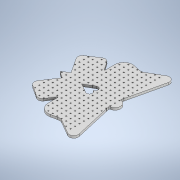
# Autodesk Inventor part: Butterfly(my own.3)
Saved by Autodesk Inventor 2020.2 (Build 242310000, 310)
## iProperties
Created: 2020-02-15
Part Number: Butterfly(my own.3)
Material: Generic
Document SubType Name: Modeling
Designer: lenovo
Density: 1 g/cm^3
Appearance: Default
Author: lenovo
Autodesk Inventor part; units mm, degrees
ref_plane "YZ Plane" through (0, 0, 0) normal (1, 0, 0) x (0, 1, 0)
ref_plane "XZ Plane" through (0, 0, 0) normal (0, 1, 0) x (-1, 0, 0)
ref_plane "XY Plane" through (0, 0, 0) normal (0, 0, 1) x (1, 0, 0)
sketch "Sketch1" plane through (0, 0, 0) normal (0, 1, 0) x (-1, 0, 0)
  line L0 (22.8541, 0.8351) -> (9.6752, 9.5184)
  line L1 (24.1214, 0.0001) -> (39.9037, 0.0001) construction
  line L2 (9.3904, 10.9036) -> (30.8478, 43.4702)
  line L3 (27.9993, 57.3225) -> (2.9481, 73.8281)
  line L4 (-10.9042, 70.9796) -> (-22.8239, 52.8887)
  line L5 (-24.659, 53.4389) -> (-24.659, 85.1036)
  line L6 (-24.659, 85.1036) -> (-24.659, 75.1841)
  line L7 (-48.9878, 94.7101) -> (-62.9353, 91.618)
  line L8 (-73.6103, 93.261) -> (-105.0047, 111.3865)
  line L9 (-119.7515, 100.4904) -> (-99.9709, 14.2618)
  line L10 (-124.8839, 122.8638) -> (0.9973, 122.8638) construction
  arc A0 (-101.2792, 12.4343) -> (-112.4983, 0.0001) centre (-99.9983, 0.0001) ccw
  line L11 (40, 0.0001) -> (-130, 0.0001)
  line L12 (22.8541, -0.8349) -> (9.6752, -9.5182)
  line L13 (9.3904, -10.9034) -> (30.8478, -43.47)
  line L14 (27.9993, -57.3223) -> (2.9481, -73.8279)
  line L15 (-10.9042, -70.9794) -> (-22.8239, -52.8885)
  line L16 (-24.659, -53.4387) -> (-24.659, -85.1034)
  line L17 (-24.659, -85.1034) -> (-24.659, -75.1839)
  line L18 (-48.9878, -94.7099) -> (-62.9353, -91.6178)
  line L19 (-73.6103, -93.2608) -> (-105.0047, -111.3864)
  line L20 (-119.7515, -100.4902) -> (-99.9709, -14.2616)
  arc A1 (-112.4983, 0.0001) -> (-101.2792, -12.4341) centre (-99.9983, 0.0001) ccw
  arc A2 (30.8478, 43.4702) -> (27.9993, 57.3225) centre (22.4974, 48.9721) ccw
  arc A3 (2.9481, 73.8281) -> (-10.9042, 70.9796) centre (-2.5538, 65.4777) ccw
  arc A4 (27.9993, -57.3223) -> (30.8478, -43.47) centre (22.4974, -48.9719) ccw
  arc A5 (-10.9042, -70.9794) -> (2.9481, -73.8279) centre (-2.5538, -65.4775) ccw
  arc A6 (-24.659, 53.4389) -> (-22.8239, 52.8887) centre (-23.659, 53.4389) ccw
  arc A7 (-22.8239, -52.8885) -> (-24.659, -53.4387) centre (-23.659, -53.4387) ccw
  arc A8 (9.3904, 10.9036) -> (9.6752, 9.5184) centre (10.2254, 10.3534) ccw
  arc A9 (9.6752, -9.5182) -> (9.3904, -10.9034) centre (10.2254, -10.3532) ccw
  arc A10 (22.8541, -0.8349) -> (22.8541, 0.8351) centre (22.3039, 0.0001) ccw
  arc A11 (-24.659, 75.1841) -> (-48.9878, 94.7101) centre (-44.659, 75.1841) ccw
  arc A12 (-48.9878, -94.7099) -> (-24.659, -75.1839) centre (-44.659, -75.1839) ccw
  arc A13 (-105.0047, 111.3865) -> (-119.7515, 100.4904) centre (-110.0047, 102.7263) ccw
  arc A14 (-119.7515, -100.4902) -> (-105.0047, -111.3864) centre (-110.0047, -102.7261) ccw
  arc A15 (-73.6103, 93.261) -> (-62.9353, 91.618) centre (-66.1603, 106.1648) ccw
  arc A16 (-62.9353, -91.6178) -> (-73.6103, -93.2608) centre (-66.1603, -106.1646) ccw
  arc A17 (-101.2792, 12.4343) -> (-99.9709, 14.2618) centre (-101.4329, 13.9264) ccw
  arc A18 (-99.9709, -14.2616) -> (-101.2792, -12.4341) centre (-101.4329, -13.9262) ccw
  point P0 (0, 0)
  point P1 (8.8402, 10.0686)
  point P2 (36.3497, 51.8206)
  point P3 (-5.4023, 79.33)
  point P4 (-24.659, 50.1036)
  point P5 (-24.659, 100.1036)
  point P6 (-68.5923, 90.3638)
  point P7 (-99.565, 12.4926)
  point P8 (8.8402, -10.0684)
  point P9 (36.3497, -51.8204)
  point P10 (-5.4023, -79.3298)
  point P11 (-24.659, -50.1034)
  point P12 (-24.659, -100.1034)
  point P13 (-68.5923, -90.3636)
  point P14 (-124.8839, -122.8636)
  point P15 (-99.565, -12.4924)
  dimension "d0" = 18.3
  dimension "d1" = 146.62
  dimension "d2" = 50
  dimension "d3" = 90
  dimension "d4" = 50
  dimension "d5" = 90
  dimension "d6" = 35
  dimension "d7" = 90
  dimension "d8" = 35
  dimension "d9" = 15
  dimension "d10" = 45
  dimension "d11" = 77.5
  dimension "d12" = 65
  dimension "d13" = 137.5
  dimension "d14" = 77.08
  dimension "d15" = 25
  dimension "d16" = 170
  dimension "d17" = 10
  dimension "d18" = 1
  dimension "d19" = 20
  dimension "d20" = 14.9
  dimension "d21" = 1.5
  constraints: 42 end point, 40 point on circle, 37 point on line, 34 tangent, 19 centre point, 12 equal radius, 9 symmetric about line, 3 perpendicular, 2 horizontal, 1 equal length, 1 vertical, 1 other
  measures "d0" distance of L1.start point (8.84, 10.069)
  measures "d1" angle of L1 L0
  measures "d2" distance of point (8.84, 10.069) point (36.35, 51.821)
  measures "d3" angle of L0 L2
  measures "d4" distance of point (36.35, 51.821) point (-5.402, 79.33)
  measures "d5" angle of L3 L2
  measures "d6" distance of point (-5.402, 79.33) point (-24.659, 50.104)
  measures "d7" angle of L4 L3
  measures "d8" distance of point (-24.659, 50.104) L5.end
  measures "d9" distance of L5.end point (-24.659, 100.104)
  measures "d10" distance of point (-24.659, 100.104) point (-68.592, 90.364)
  measures "d11" angle of L7 L6
  measures "d12" distance of point (-68.592, 90.364) L10.start
  measures "d13" angle of L7 L8
  measures "d14" angle of L9 L10
  measures "d15" diameter of A0
  measures "d16" distance of L11.start L11.end
  measures "d17" radius of A2
  measures "d18" radius of A6
  measures "d19" radius of A11
  measures "d20" radius of A15
  measures "d21" radius of A17
extrude "Extrusion1" add sketch "Sketch1" along normal blind 5
sketch "Sketch2" plane through (0, 5, 0) normal (0, 1, 0) x (1, 0, 0)
  line L0 (-1, -1) -> (1, -1)
  line L1 (1, -1) -> (1, 1)
  line L2 (1, 1) -> (-1, 1)
  line L3 (-1, 1) -> (-1, -1)
  line L4 (-1, -1) -> (1, 1) construction
  line L5 (1, -1) -> (-1, 1) construction
  line L6 (-55, 0) -> (141.5585, 0)
  line L7 (0, 115) -> (0, -134.2875)
  line L8 (11, 1) -> (9, 1)
  line L9 (9, 1) -> (9, -1)
  line L10 (11, -1) -> (11, 1)
  line L11 (9, -1) -> (11, -1)
  line L12 (21, 1) -> (19, 1)
  line L13 (19, 1) -> (19, -1)
  line L14 (21, -1) -> (21, 1)
  line L15 (19, -1) -> (21, -1)
  line L16 (31, 1) -> (29, 1)
  line L17 (29, 1) -> (29, -1)
  line L18 (31, -1) -> (31, 1)
  line L19 (29, -1) -> (31, -1)
  line L20 (41, 1) -> (39, 1)
  line L21 (39, 1) -> (39, -1)
  line L22 (41, -1) -> (41, 1)
  line L23 (39, -1) -> (41, -1)
  line L24 (51, 1) -> (49, 1)
  line L25 (49, 1) -> (49, -1)
  line L26 (51, -1) -> (51, 1)
  line L27 (49, -1) -> (51, -1)
  line L28 (61, 1) -> (59, 1)
  line L29 (59, 1) -> (59, -1)
  line L30 (61, -1) -> (61, 1)
  line L31 (59, -1) -> (61, -1)
  line L32 (71, 1) -> (69, 1)
  line L33 (69, 1) -> (69, -1)
  line L34 (71, -1) -> (71, 1)
  line L35 (69, -1) -> (71, -1)
  line L36 (81, 1) -> (79, 1)
  line L37 (79, 1) -> (79, -1)
  line L38 (81, -1) -> (81, 1)
  line L39 (79, -1) -> (81, -1)
  line L40 (91, 1) -> (89, 1)
  line L41 (89, 1) -> (89, -1)
  line L42 (91, -1) -> (91, 1)
  line L43 (89, -1) -> (91, -1)
  line L44 (101, 1) -> (99, 1)
  line L45 (99, 1) -> (99, -1)
  line L46 (101, -1) -> (101, 1)
  line L47 (99, -1) -> (101, -1)
  line L48 (1, -9) -> (-1, -9)
  line L49 (-1, -9) -> (-1, -11)
  line L50 (1, -11) -> (1, -9)
  line L51 (-1, -11) -> (1, -11)
  line L52 (11, -9) -> (9, -9)
  line L53 (9, -9) -> (9, -11)
  line L54 (11, -11) -> (11, -9)
  line L55 (9, -11) -> (11, -11)
  line L56 (21, -9) -> (19, -9)
  line L57 (19, -9) -> (19, -11)
  line L58 (21, -11) -> (21, -9)
  line L59 (19, -11) -> (21, -11)
  line L60 (31, -9) -> (29, -9)
  line L61 (29, -9) -> (29, -11)
  line L62 (31, -11) -> (31, -9)
  line L63 (29, -11) -> (31, -11)
  line L64 (41, -9) -> (39, -9)
  line L65 (39, -9) -> (39, -11)
  line L66 (41, -11) -> (41, -9)
  line L67 (39, -11) -> (41, -11)
  line L68 (51, -9) -> (49, -9)
  line L69 (49, -9) -> (49, -11)
  line L70 (51, -11) -> (51, -9)
  line L71 (49, -11) -> (51, -11)
  line L72 (61, -9) -> (59, -9)
  line L73 (59, -9) -> (59, -11)
  line L74 (61, -11) -> (61, -9)
  line L75 (59, -11) -> (61, -11)
  line L76 (71, -9) -> (69, -9)
  line L77 (69, -9) -> (69, -11)
  line L78 (71, -11) -> (71, -9)
  line L79 (69, -11) -> (71, -11)
  line L80 (81, -9) -> (79, -9)
  line L81 (79, -9) -> (79, -11)
  line L82 (81, -11) -> (81, -9)
  line L83 (79, -11) -> (81, -11)
  line L84 (91, -9) -> (89, -9)
  line L85 (89, -9) -> (89, -11)
  line L86 (91, -11) -> (91, -9)
  line L87 (89, -11) -> (91, -11)
  line L88 (101, -9) -> (99, -9)
  line L89 (99, -9) -> (99, -11)
  line L90 (101, -11) -> (101, -9)
  line L91 (99, -11) -> (101, -11)
  line L92 (1, -19) -> (-1, -19)
  line L93 (-1, -19) -> (-1, -21)
  line L94 (1, -21) -> (1, -19)
  line L95 (-1, -21) -> (1, -21)
  line L96 (11, -19) -> (9, -19)
  line L97 (9, -19) -> (9, -21)
  line L98 (11, -21) -> (11, -19)
  line L99 (9, -21) -> (11, -21)
  line L100 (21, -19) -> (19, -19)
  line L101 (19, -19) -> (19, -21)
  line L102 (21, -21) -> (21, -19)
  line L103 (19, -21) -> (21, -21)
  line L104 (31, -19) -> (29, -19)
  line L105 (29, -19) -> (29, -21)
  line L106 (31, -21) -> (31, -19)
  line L107 (29, -21) -> (31, -21)
  line L108 (41, -19) -> (39, -19)
  line L109 (39, -19) -> (39, -21)
  line L110 (41, -21) -> (41, -19)
  line L111 (39, -21) -> (41, -21)
  line L112 (51, -19) -> (49, -19)
  line L113 (49, -19) -> (49, -21)
  line L114 (51, -21) -> (51, -19)
  line L115 (49, -21) -> (51, -21)
  line L116 (61, -19) -> (59, -19)
  line L117 (59, -19) -> (59, -21)
  line L118 (61, -21) -> (61, -19)
  line L119 (59, -21) -> (61, -21)
  line L120 (71, -19) -> (69, -19)
  line L121 (69, -19) -> (69, -21)
  line L122 (71, -21) -> (71, -19)
  line L123 (69, -21) -> (71, -21)
  line L124 (81, -19) -> (79, -19)
  line L125 (79, -19) -> (79, -21)
  line L126 (81, -21) -> (81, -19)
  line L127 (79, -21) -> (81, -21)
  line L128 (91, -19) -> (89, -19)
  line L129 (89, -19) -> (89, -21)
  line L130 (91, -21) -> (91, -19)
  line L131 (89, -21) -> (91, -21)
  line L132 (101, -19) -> (99, -19)
  line L133 (99, -19) -> (99, -21)
  line L134 (101, -21) -> (101, -19)
  line L135 (99, -21) -> (101, -21)
  line L136 (1, -29) -> (-1, -29)
  line L137 (-1, -29) -> (-1, -31)
  line L138 (1, -31) -> (1, -29)
  line L139 (-1, -31) -> (1, -31)
  line L140 (11, -29) -> (9, -29)
  line L141 (9, -29) -> (9, -31)
  line L142 (11, -31) -> (11, -29)
  line L143 (9, -31) -> (11, -31)
  line L144 (21, -29) -> (19, -29)
  line L145 (19, -29) -> (19, -31)
  line L146 (21, -31) -> (21, -29)
  line L147 (19, -31) -> (21, -31)
  line L148 (31, -29) -> (29, -29)
  line L149 (29, -29) -> (29, -31)
  line L150 (31, -31) -> (31, -29)
  line L151 (29, -31) -> (31, -31)
  line L152 (41, -29) -> (39, -29)
  line L153 (39, -29) -> (39, -31)
  line L154 (41, -31) -> (41, -29)
  line L155 (39, -31) -> (41, -31)
  line L156 (51, -29) -> (49, -29)
  line L157 (49, -29) -> (49, -31)
  line L158 (51, -31) -> (51, -29)
  line L159 (49, -31) -> (51, -31)
  line L160 (61, -29) -> (59, -29)
  line L161 (59, -29) -> (59, -31)
  line L162 (61, -31) -> (61, -29)
  line L163 (59, -31) -> (61, -31)
  line L164 (71, -29) -> (69, -29)
  line L165 (69, -29) -> (69, -31)
  line L166 (71, -31) -> (71, -29)
  line L167 (69, -31) -> (71, -31)
  line L168 (81, -29) -> (79, -29)
  line L169 (79, -29) -> (79, -31)
  line L170 (81, -31) -> (81, -29)
  line L171 (79, -31) -> (81, -31)
  line L172 (91, -29) -> (89, -29)
  line L173 (89, -29) -> (89, -31)
  line L174 (91, -31) -> (91, -29)
  line L175 (89, -31) -> (91, -31)
  line L176 (101, -29) -> (99, -29)
  line L177 (99, -29) -> (99, -31)
  line L178 (101, -31) -> (101, -29)
  line L179 (99, -31) -> (101, -31)
  line L180 (1, -39) -> (-1, -39)
  line L181 (-1, -39) -> (-1, -41)
  line L182 (1, -41) -> (1, -39)
  line L183 (-1, -41) -> (1, -41)
  line L184 (11, -39) -> (9, -39)
  line L185 (9, -39) -> (9, -41)
  line L186 (11, -41) -> (11, -39)
  line L187 (9, -41) -> (11, -41)
  line L188 (21, -39) -> (19, -39)
  line L189 (19, -39) -> (19, -41)
  line L190 (21, -41) -> (21, -39)
  line L191 (19, -41) -> (21, -41)
  line L192 (31, -39) -> (29, -39)
  line L193 (29, -39) -> (29, -41)
  line L194 (31, -41) -> (31, -39)
  line L195 (29, -41) -> (31, -41)
  line L196 (41, -39) -> (39, -39)
  line L197 (39, -39) -> (39, -41)
  line L198 (41, -41) -> (41, -39)
  line L199 (39, -41) -> (41, -41)
  line L200 (51, -39) -> (49, -39)
  line L201 (49, -39) -> (49, -41)
  line L202 (51, -41) -> (51, -39)
  line L203 (49, -41) -> (51, -41)
  line L204 (61, -39) -> (59, -39)
  line L205 (59, -39) -> (59, -41)
  line L206 (61, -41) -> (61, -39)
  line L207 (59, -41) -> (61, -41)
  line L208 (71, -39) -> (69, -39)
  line L209 (69, -39) -> (69, -41)
  line L210 (71, -41) -> (71, -39)
  line L211 (69, -41) -> (71, -41)
  line L212 (81, -39) -> (79, -39)
  line L213 (79, -39) -> (79, -41)
  line L214 (81, -41) -> (81, -39)
  line L215 (79, -41) -> (81, -41)
  line L216 (91, -39) -> (89, -39)
  line L217 (89, -39) -> (89, -41)
  line L218 (91, -41) -> (91, -39)
  line L219 (89, -41) -> (91, -41)
  line L220 (101, -39) -> (99, -39)
  line L221 (99, -39) -> (99, -41)
  line L222 (101, -41) -> (101, -39)
  line L223 (99, -41) -> (101, -41)
  line L224 (1, -49) -> (-1, -49)
  line L225 (-1, -49) -> (-1, -51)
  line L226 (1, -51) -> (1, -49)
  line L227 (-1, -51) -> (1, -51)
  line L228 (11, -49) -> (9, -49)
  line L229 (9, -49) -> (9, -51)
  line L230 (11, -51) -> (11, -49)
  line L231 (9, -51) -> (11, -51)
  line L232 (21, -49) -> (19, -49)
  line L233 (19, -49) -> (19, -51)
  line L234 (21, -51) -> (21, -49)
  line L235 (19, -51) -> (21, -51)
  line L236 (31, -49) -> (29, -49)
  line L237 (29, -49) -> (29, -51)
  line L238 (31, -51) -> (31, -49)
  line L239 (29, -51) -> (31, -51)
  line L240 (41, -49) -> (39, -49)
  line L241 (39, -49) -> (39, -51)
  line L242 (41, -51) -> (41, -49)
  line L243 (39, -51) -> (41, -51)
  line L244 (51, -49) -> (49, -49)
  line L245 (49, -49) -> (49, -51)
  line L246 (51, -51) -> (51, -49)
  line L247 (49, -51) -> (51, -51)
  line L248 (61, -49) -> (59, -49)
  line L249 (59, -49) -> (59, -51)
  line L250 (61, -51) -> (61, -49)
  line L251 (59, -51) -> (61, -51)
  line L252 (71, -49) -> (69, -49)
  line L253 (69, -49) -> (69, -51)
  line L254 (71, -51) -> (71, -49)
  line L255 (69, -51) -> (71, -51)
  line L256 (81, -49) -> (79, -49)
  line L257 (79, -49) -> (79, -51)
  line L258 (81, -51) -> (81, -49)
  line L259 (79, -51) -> (81, -51)
  line L260 (91, -49) -> (89, -49)
  line L261 (89, -49) -> (89, -51)
  line L262 (91, -51) -> (91, -49)
  line L263 (89, -51) -> (91, -51)
  line L264 (101, -49) -> (99, -49)
  line L265 (99, -49) -> (99, -51)
  line L266 (101, -51) -> (101, -49)
  line L267 (99, -51) -> (101, -51)
  line L268 (1, -59) -> (-1, -59)
  line L269 (-1, -59) -> (-1, -61)
  line L270 (1, -61) -> (1, -59)
  line L271 (-1, -61) -> (1, -61)
  line L272 (11, -59) -> (9, -59)
  line L273 (9, -59) -> (9, -61)
  line L274 (11, -61) -> (11, -59)
  line L275 (9, -61) -> (11, -61)
  line L276 (21, -59) -> (19, -59)
  line L277 (19, -59) -> (19, -61)
  line L278 (21, -61) -> (21, -59)
  line L279 (19, -61) -> (21, -61)
  line L280 (31, -59) -> (29, -59)
  line L281 (29, -59) -> (29, -61)
  line L282 (31, -61) -> (31, -59)
  line L283 (29, -61) -> (31, -61)
  line L284 (41, -59) -> (39, -59)
  line L285 (39, -59) -> (39, -61)
  line L286 (41, -61) -> (41, -59)
  line L287 (39, -61) -> (41, -61)
  line L288 (51, -59) -> (49, -59)
  line L289 (49, -59) -> (49, -61)
  line L290 (51, -61) -> (51, -59)
  line L291 (49, -61) -> (51, -61)
  line L292 (61, -59) -> (59, -59)
  line L293 (59, -59) -> (59, -61)
  line L294 (61, -61) -> (61, -59)
  line L295 (59, -61) -> (61, -61)
  line L296 (71, -59) -> (69, -59)
  line L297 (69, -59) -> (69, -61)
  line L298 (71, -61) -> (71, -59)
  line L299 (69, -61) -> (71, -61)
  line L300 (81, -59) -> (79, -59)
  line L301 (79, -59) -> (79, -61)
  line L302 (81, -61) -> (81, -59)
  line L303 (79, -61) -> (81, -61)
  line L304 (91, -59) -> (89, -59)
  line L305 (89, -59) -> (89, -61)
  line L306 (91, -61) -> (91, -59)
  line L307 (89, -61) -> (91, -61)
  line L308 (101, -59) -> (99, -59)
  line L309 (99, -59) -> (99, -61)
  line L310 (101, -61) -> (101, -59)
  line L311 (99, -61) -> (101, -61)
  line L312 (1, -69) -> (-1, -69)
  line L313 (-1, -69) -> (-1, -71)
  line L314 (1, -71) -> (1, -69)
  line L315 (-1, -71) -> (1, -71)
  line L316 (11, -69) -> (9, -69)
  line L317 (9, -69) -> (9, -71)
  line L318 (11, -71) -> (11, -69)
  line L319 (9, -71) -> (11, -71)
  line L320 (21, -69) -> (19, -69)
  line L321 (19, -69) -> (19, -71)
  line L322 (21, -71) -> (21, -69)
  line L323 (19, -71) -> (21, -71)
  line L324 (31, -69) -> (29, -69)
  line L325 (29, -69) -> (29, -71)
  line L326 (31, -71) -> (31, -69)
  line L327 (29, -71) -> (31, -71)
  line L328 (41, -69) -> (39, -69)
  line L329 (39, -69) -> (39, -71)
  line L330 (41, -71) -> (41, -69)
  line L331 (39, -71) -> (41, -71)
  line L332 (51, -69) -> (49, -69)
  line L333 (49, -69) -> (49, -71)
  line L334 (51, -71) -> (51, -69)
  line L335 (49, -71) -> (51, -71)
  line L336 (61, -69) -> (59, -69)
  line L337 (59, -69) -> (59, -71)
  line L338 (61, -71) -> (61, -69)
  line L339 (59, -71) -> (61, -71)
  line L340 (71, -69) -> (69, -69)
  line L341 (69, -69) -> (69, -71)
  line L342 (71, -71) -> (71, -69)
  line L343 (69, -71) -> (71, -71)
  line L344 (81, -69) -> (79, -69)
  line L345 (79, -69) -> (79, -71)
  line L346 (81, -71) -> (81, -69)
  line L347 (79, -71) -> (81, -71)
  line L348 (91, -69) -> (89, -69)
  line L349 (89, -69) -> (89, -71)
  line L350 (91, -71) -> (91, -69)
  line L351 (89, -71) -> (91, -71)
  line L352 (101, -69) -> (99, -69)
  line L353 (99, -69) -> (99, -71)
  line L354 (101, -71) -> (101, -69)
  line L355 (99, -71) -> (101, -71)
  line L356 (1, -79) -> (-1, -79)
  line L357 (-1, -79) -> (-1, -81)
  line L358 (1, -81) -> (1, -79)
  line L359 (-1, -81) -> (1, -81)
  line L360 (11, -79) -> (9, -79)
  line L361 (9, -79) -> (9, -81)
  line L362 (11, -81) -> (11, -79)
  line L363 (9, -81) -> (11, -81)
  line L364 (21, -79) -> (19, -79)
  line L365 (19, -79) -> (19, -81)
  line L366 (21, -81) -> (21, -79)
  line L367 (19, -81) -> (21, -81)
  line L368 (31, -79) -> (29, -79)
  line L369 (29, -79) -> (29, -81)
  line L370 (31, -81) -> (31, -79)
  line L371 (29, -81) -> (31, -81)
  line L372 (41, -79) -> (39, -79)
  line L373 (39, -79) -> (39, -81)
  line L374 (41, -81) -> (41, -79)
  line L375 (39, -81) -> (41, -81)
  line L376 (51, -79) -> (49, -79)
  line L377 (49, -79) -> (49, -81)
  line L378 (51, -81) -> (51, -79)
  line L379 (49, -81) -> (51, -81)
  line L380 (61, -79) -> (59, -79)
  line L381 (59, -79) -> (59, -81)
  line L382 (61, -81) -> (61, -79)
  line L383 (59, -81) -> (61, -81)
  line L384 (71, -79) -> (69, -79)
  line L385 (69, -79) -> (69, -81)
  line L386 (71, -81) -> (71, -79)
  line L387 (69, -81) -> (71, -81)
  line L388 (81, -79) -> (79, -79)
  line L389 (79, -79) -> (79, -81)
  line L390 (81, -81) -> (81, -79)
  line L391 (79, -81) -> (81, -81)
  line L392 (91, -79) -> (89, -79)
  line L393 (89, -79) -> (89, -81)
  line L394 (91, -81) -> (91, -79)
  line L395 (89, -81) -> (91, -81)
  line L396 (101, -79) -> (99, -79)
  line L397 (99, -79) -> (99, -81)
  line L398 (101, -81) -> (101, -79)
  line L399 (99, -81) -> (101, -81)
  line L400 (1, -89) -> (-1, -89)
  line L401 (-1, -89) -> (-1, -91)
  line L402 (1, -91) -> (1, -89)
  line L403 (-1, -91) -> (1, -91)
  line L404 (11, -89) -> (9, -89)
  line L405 (9, -89) -> (9, -91)
  line L406 (11, -91) -> (11, -89)
  line L407 (9, -91) -> (11, -91)
  line L408 (21, -89) -> (19, -89)
  line L409 (19, -89) -> (19, -91)
  line L410 (21, -91) -> (21, -89)
  line L411 (19, -91) -> (21, -91)
  line L412 (31, -89) -> (29, -89)
  line L413 (29, -89) -> (29, -91)
  line L414 (31, -91) -> (31, -89)
  line L415 (29, -91) -> (31, -91)
  line L416 (41, -89) -> (39, -89)
  line L417 (39, -89) -> (39, -91)
  line L418 (41, -91) -> (41, -89)
  line L419 (39, -91) -> (41, -91)
  line L420 (51, -89) -> (49, -89)
  line L421 (49, -89) -> (49, -91)
  line L422 (51, -91) -> (51, -89)
  line L423 (49, -91) -> (51, -91)
  line L424 (61, -89) -> (59, -89)
  line L425 (59, -89) -> (59, -91)
  line L426 (61, -91) -> (61, -89)
  line L427 (59, -91) -> (61, -91)
  line L428 (71, -89) -> (69, -89)
  line L429 (69, -89) -> (69, -91)
  line L430 (71, -91) -> (71, -89)
  line L431 (69, -91) -> (71, -91)
  line L432 (81, -89) -> (79, -89)
  line L433 (79, -89) -> (79, -91)
  line L434 (81, -91) -> (81, -89)
  line L435 (79, -91) -> (81, -91)
  line L436 (91, -89) -> (89, -89)
  line L437 (89, -89) -> (89, -91)
  line L438 (91, -91) -> (91, -89)
  line L439 (89, -91) -> (91, -91)
  line L440 (101, -89) -> (99, -89)
  line L441 (99, -89) -> (99, -91)
  line L442 (101, -91) -> (101, -89)
  line L443 (99, -91) -> (101, -91)
  line L444 (1, -99) -> (-1, -99)
  line L445 (-1, -99) -> (-1, -101)
  line L446 (1, -101) -> (1, -99)
  line L447 (-1, -101) -> (1, -101)
  line L448 (11, -99) -> (9, -99)
  line L449 (9, -99) -> (9, -101)
  line L450 (11, -101) -> (11, -99)
  line L451 (9, -101) -> (11, -101)
  line L452 (21, -99) -> (19, -99)
  line L453 (19, -99) -> (19, -101)
  line L454 (21, -101) -> (21, -99)
  line L455 (19, -101) -> (21, -101)
  line L456 (31, -99) -> (29, -99)
  line L457 (29, -99) -> (29, -101)
  line L458 (31, -101) -> (31, -99)
  line L459 (29, -101) -> (31, -101)
  line L460 (41, -99) -> (39, -99)
  line L461 (39, -99) -> (39, -101)
  line L462 (41, -101) -> (41, -99)
  line L463 (39, -101) -> (41, -101)
  line L464 (51, -99) -> (49, -99)
  line L465 (49, -99) -> (49, -101)
  line L466 (51, -101) -> (51, -99)
  line L467 (49, -101) -> (51, -101)
  line L468 (61, -99) -> (59, -99)
  line L469 (59, -99) -> (59, -101)
  line L470 (61, -101) -> (61, -99)
  line L471 (59, -101) -> (61, -101)
  line L472 (71, -99) -> (69, -99)
  line L473 (69, -99) -> (69, -101)
  line L474 (71, -101) -> (71, -99)
  line L475 (69, -101) -> (71, -101)
  line L476 (81, -99) -> (79, -99)
  line L477 (79, -99) -> (79, -101)
  line L478 (81, -101) -> (81, -99)
  line L479 (79, -101) -> (81, -101)
  line L480 (91, -99) -> (89, -99)
  line L481 (89, -99) -> (89, -101)
  line L482 (91, -101) -> (91, -99)
  line L483 (89, -101) -> (91, -101)
  line L484 (101, -99) -> (99, -99)
  line L485 (99, -99) -> (99, -101)
  line L486 (101, -101) -> (101, -99)
  line L487 (99, -101) -> (101, -101)
  line L488 (51, 1) -> (49, 1)
  line L489 (49, 1) -> (49, -1)
  line L490 (49, -1) -> (51, -1)
  line L491 (61, 1) -> (59, 1)
  line L492 (59, -1) -> (61, -1)
  line L493 (61, -1) -> (61, 1)
  line L494 (59, 1) -> (59, -1)
  line L495 (51, -1) -> (51, 1)
  line L496 (31, 1) -> (29, 1)
  line L497 (29, 1) -> (29, -1)
  line L498 (29, -1) -> (31, -1)
  line L499 (31, -1) -> (31, 1)
  line L500 (41, 1) -> (39, 1)
  line L501 (39, 1) -> (39, -1)
  line L502 (41, -1) -> (41, 1)
  line L503 (39, -1) -> (41, -1)
  line L504 (71, 1) -> (69, 1)
  line L505 (69, 1) -> (69, -1)
  line L506 (71, -1) -> (71, 1)
  line L507 (69, -1) -> (71, -1)
  line L508 (79, -1) -> (81, -1)
  line L509 (79, 1) -> (79, -1)
  line L510 (81, -1) -> (81, 1)
  line L511 (81, 1) -> (79, 1)
  line L512 (91, 1) -> (89, 1)
  line L513 (89, 1) -> (89, -1)
  line L514 (91, -1) -> (91, 1)
  line L515 (89, -1) -> (91, -1)
  line L516 (99, -1) -> (101, -1)
  line L517 (99, 1) -> (99, -1)
  line L518 (101, -1) -> (101, 1)
  line L519 (101, 1) -> (99, 1)
  line L520 (11, 1) -> (9, 1)
  line L521 (1, 1) -> (-1, 1)
  line L522 (1, -1) -> (1, 1)
  line L523 (9, 1) -> (9, -1)
  line L524 (11, -1) -> (11, 1)
  line L525 (9, -1) -> (11, -1)
  line L526 (-1, 1) -> (-1, -1)
  line L527 (-1, -1) -> (1, -1)
  line L528 (21, 1) -> (19, 1)
  line L529 (19, 1) -> (19, -1)
  line L530 (21, -1) -> (21, 1)
  line L531 (19, -1) -> (21, -1)
  line L532 (0, 125) -> (0, -124.2875)
  line L533 (51, 11) -> (49, 11)
  line L534 (49, 11) -> (49, 9)
  line L535 (49, 9) -> (51, 9)
  line L536 (61, 11) -> (59, 11)
  line L537 (59, 9) -> (61, 9)
  line L538 (61, 9) -> (61, 11)
  line L539 (59, 11) -> (59, 9)
  line L540 (51, 9) -> (51, 11)
  line L541 (31, 11) -> (29, 11)
  line L542 (29, 11) -> (29, 9)
  line L543 (29, 9) -> (31, 9)
  line L544 (31, 9) -> (31, 11)
  line L545 (41, 11) -> (39, 11)
  line L546 (39, 11) -> (39, 9)
  line L547 (41, 9) -> (41, 11)
  line L548 (39, 9) -> (41, 9)
  line L549 (71, 11) -> (69, 11)
  line L550 (69, 11) -> (69, 9)
  line L551 (71, 9) -> (71, 11)
  line L552 (69, 9) -> (71, 9)
  line L553 (79, 9) -> (81, 9)
  line L554 (79, 11) -> (79, 9)
  line L555 (81, 9) -> (81, 11)
  line L556 (81, 11) -> (79, 11)
  line L557 (91, 11) -> (89, 11)
  line L558 (89, 11) -> (89, 9)
  line L559 (91, 9) -> (91, 11)
  line L560 (89, 9) -> (91, 9)
  line L561 (99, 9) -> (101, 9)
  line L562 (99, 11) -> (99, 9)
  line L563 (101, 9) -> (101, 11)
  line L564 (101, 11) -> (99, 11)
  line L565 (11, 11) -> (9, 11)
  line L566 (1, 11) -> (-1, 11)
  line L567 (1, 9) -> (1, 11)
  line L568 (9, 11) -> (9, 9)
  line L569 (11, 9) -> (11, 11)
  line L570 (9, 9) -> (11, 9)
  line L571 (-1, 11) -> (-1, 9)
  line L572 (-1, 9) -> (1, 9)
  line L573 (21, 11) -> (19, 11)
  line L574 (19, 11) -> (19, 9)
  line L575 (21, 9) -> (21, 11)
  line L576 (19, 9) -> (21, 9)
  line L577 (0, 135) -> (0, -114.2875)
  line L578 (51, 21) -> (49, 21)
  line L579 (49, 21) -> (49, 19)
  line L580 (49, 19) -> (51, 19)
  line L581 (61, 21) -> (59, 21)
  line L582 (59, 19) -> (61, 19)
  line L583 (61, 19) -> (61, 21)
  line L584 (59, 21) -> (59, 19)
  line L585 (51, 19) -> (51, 21)
  line L586 (31, 21) -> (29, 21)
  line L587 (29, 21) -> (29, 19)
  line L588 (29, 19) -> (31, 19)
  line L589 (31, 19) -> (31, 21)
  line L590 (41, 21) -> (39, 21)
  line L591 (39, 21) -> (39, 19)
  line L592 (41, 19) -> (41, 21)
  line L593 (39, 19) -> (41, 19)
  line L594 (71, 21) -> (69, 21)
  line L595 (69, 21) -> (69, 19)
  line L596 (71, 19) -> (71, 21)
  line L597 (69, 19) -> (71, 19)
  line L598 (79, 19) -> (81, 19)
  line L599 (79, 21) -> (79, 19)
  line L600 (81, 19) -> (81, 21)
  line L601 (81, 21) -> (79, 21)
  line L602 (91, 21) -> (89, 21)
  line L603 (89, 21) -> (89, 19)
  line L604 (91, 19) -> (91, 21)
  line L605 (89, 19) -> (91, 19)
  line L606 (99, 19) -> (101, 19)
  line L607 (99, 21) -> (99, 19)
  line L608 (101, 19) -> (101, 21)
  line L609 (101, 21) -> (99, 21)
  line L610 (11, 21) -> (9, 21)
  line L611 (1, 21) -> (-1, 21)
  line L612 (1, 19) -> (1, 21)
  line L613 (9, 21) -> (9, 19)
  line L614 (11, 19) -> (11, 21)
  line L615 (9, 19) -> (11, 19)
  line L616 (-1, 21) -> (-1, 19)
  line L617 (-1, 19) -> (1, 19)
  line L618 (21, 21) -> (19, 21)
  line L619 (19, 21) -> (19, 19)
  line L620 (21, 19) -> (21, 21)
  line L621 (19, 19) -> (21, 19)
  line L622 (0, 145) -> (0, -104.2875)
  line L623 (51, 31) -> (49, 31)
  line L624 (49, 31) -> (49, 29)
  line L625 (49, 29) -> (51, 29)
  line L626 (61, 31) -> (59, 31)
  line L627 (59, 29) -> (61, 29)
  line L628 (61, 29) -> (61, 31)
  line L629 (59, 31) -> (59, 29)
  line L630 (51, 29) -> (51, 31)
  line L631 (31, 31) -> (29, 31)
  line L632 (29, 31) -> (29, 29)
  line L633 (29, 29) -> (31, 29)
  line L634 (31, 29) -> (31, 31)
  line L635 (41, 31) -> (39, 31)
  line L636 (39, 31) -> (39, 29)
  line L637 (41, 29) -> (41, 31)
  line L638 (39, 29) -> (41, 29)
  line L639 (71, 31) -> (69, 31)
  line L640 (69, 31) -> (69, 29)
  line L641 (71, 29) -> (71, 31)
  line L642 (69, 29) -> (71, 29)
  line L643 (79, 29) -> (81, 29)
  line L644 (79, 31) -> (79, 29)
  line L645 (81, 29) -> (81, 31)
  line L646 (81, 31) -> (79, 31)
  line L647 (91, 31) -> (89, 31)
  line L648 (89, 31) -> (89, 29)
  line L649 (91, 29) -> (91, 31)
  line L650 (89, 29) -> (91, 29)
  line L651 (99, 29) -> (101, 29)
  line L652 (99, 31) -> (99, 29)
  line L653 (101, 29) -> (101, 31)
  line L654 (101, 31) -> (99, 31)
  line L655 (11, 31) -> (9, 31)
  line L656 (1, 31) -> (-1, 31)
  line L657 (1, 29) -> (1, 31)
  line L658 (9, 31) -> (9, 29)
  line L659 (11, 29) -> (11, 31)
  line L660 (9, 29) -> (11, 29)
  line L661 (-1, 31) -> (-1, 29)
  line L662 (-1, 29) -> (1, 29)
  line L663 (21, 31) -> (19, 31)
  line L664 (19, 31) -> (19, 29)
  line L665 (21, 29) -> (21, 31)
  line L666 (19, 29) -> (21, 29)
  line L667 (0, 155) -> (0, -94.2875)
  line L668 (51, 41) -> (49, 41)
  line L669 (49, 41) -> (49, 39)
  line L670 (49, 39) -> (51, 39)
  line L671 (61, 41) -> (59, 41)
  line L672 (59, 39) -> (61, 39)
  line L673 (61, 39) -> (61, 41)
  line L674 (59, 41) -> (59, 39)
  line L675 (51, 39) -> (51, 41)
  line L676 (31, 41) -> (29, 41)
  line L677 (29, 41) -> (29, 39)
  line L678 (29, 39) -> (31, 39)
  line L679 (31, 39) -> (31, 41)
  line L680 (41, 41) -> (39, 41)
  line L681 (39, 41) -> (39, 39)
  line L682 (41, 39) -> (41, 41)
  line L683 (39, 39) -> (41, 39)
  line L684 (71, 41) -> (69, 41)
  line L685 (69, 41) -> (69, 39)
  line L686 (71, 39) -> (71, 41)
  line L687 (69, 39) -> (71, 39)
  line L688 (79, 39) -> (81, 39)
  line L689 (79, 41) -> (79, 39)
  line L690 (81, 39) -> (81, 41)
  line L691 (81, 41) -> (79, 41)
  line L692 (91, 41) -> (89, 41)
  line L693 (89, 41) -> (89, 39)
  line L694 (91, 39) -> (91, 41)
  line L695 (89, 39) -> (91, 39)
  line L696 (99, 39) -> (101, 39)
  line L697 (99, 41) -> (99, 39)
  line L698 (101, 39) -> (101, 41)
  line L699 (101, 41) -> (99, 41)
  line L700 (11, 41) -> (9, 41)
  line L701 (1, 41) -> (-1, 41)
  line L702 (1, 39) -> (1, 41)
  line L703 (9, 41) -> (9, 39)
  line L704 (11, 39) -> (11, 41)
  line L705 (9, 39) -> (11, 39)
  line L706 (-1, 41) -> (-1, 39)
  line L707 (-1, 39) -> (1, 39)
  line L708 (21, 41) -> (19, 41)
  line L709 (19, 41) -> (19, 39)
  line L710 (21, 39) -> (21, 41)
  line L711 (19, 39) -> (21, 39)
  line L712 (0, 165) -> (0, -84.2875)
  line L713 (51, 51) -> (49, 51)
  line L714 (49, 51) -> (49, 49)
  line L715 (49, 49) -> (51, 49)
  line L716 (61, 51) -> (59, 51)
  line L717 (59, 49) -> (61, 49)
  line L718 (61, 49) -> (61, 51)
  line L719 (59, 51) -> (59, 49)
  line L720 (51, 49) -> (51, 51)
  line L721 (31, 51) -> (29, 51)
  line L722 (29, 51) -> (29, 49)
  line L723 (29, 49) -> (31, 49)
  line L724 (31, 49) -> (31, 51)
  line L725 (41, 51) -> (39, 51)
  line L726 (39, 51) -> (39, 49)
  line L727 (41, 49) -> (41, 51)
  line L728 (39, 49) -> (41, 49)
  line L729 (71, 51) -> (69, 51)
  line L730 (69, 51) -> (69, 49)
  line L731 (71, 49) -> (71, 51)
  line L732 (69, 49) -> (71, 49)
  line L733 (79, 49) -> (81, 49)
  line L734 (79, 51) -> (79, 49)
  line L735 (81, 49) -> (81, 51)
  line L736 (81, 51) -> (79, 51)
  line L737 (91, 51) -> (89, 51)
  line L738 (89, 51) -> (89, 49)
  line L739 (91, 49) -> (91, 51)
  line L740 (89, 49) -> (91, 49)
  line L741 (99, 49) -> (101, 49)
  line L742 (99, 51) -> (99, 49)
  line L743 (101, 49) -> (101, 51)
  line L744 (101, 51) -> (99, 51)
  line L745 (11, 51) -> (9, 51)
  line L746 (1, 51) -> (-1, 51)
  line L747 (1, 49) -> (1, 51)
  line L748 (9, 51) -> (9, 49)
  line L749 (11, 49) -> (11, 51)
  line L750 (9, 49) -> (11, 49)
  line L751 (-1, 51) -> (-1, 49)
  line L752 (-1, 49) -> (1, 49)
  line L753 (21, 51) -> (19, 51)
  line L754 (19, 51) -> (19, 49)
  line L755 (21, 49) -> (21, 51)
  line L756 (19, 49) -> (21, 49)
  line L757 (0, 175) -> (0, -74.2875)
  line L758 (51, 61) -> (49, 61)
  line L759 (49, 61) -> (49, 59)
  line L760 (49, 59) -> (51, 59)
  line L761 (61, 61) -> (59, 61)
  line L762 (59, 59) -> (61, 59)
  line L763 (61, 59) -> (61, 61)
  line L764 (59, 61) -> (59, 59)
  line L765 (51, 59) -> (51, 61)
  line L766 (31, 61) -> (29, 61)
  line L767 (29, 61) -> (29, 59)
  line L768 (29, 59) -> (31, 59)
  line L769 (31, 59) -> (31, 61)
  line L770 (41, 61) -> (39, 61)
  line L771 (39, 61) -> (39, 59)
  line L772 (41, 59) -> (41, 61)
  line L773 (39, 59) -> (41, 59)
  line L774 (71, 61) -> (69, 61)
  line L775 (69, 61) -> (69, 59)
  line L776 (71, 59) -> (71, 61)
  line L777 (69, 59) -> (71, 59)
  line L778 (79, 59) -> (81, 59)
  line L779 (79, 61) -> (79, 59)
  line L780 (81, 59) -> (81, 61)
  line L781 (81, 61) -> (79, 61)
  line L782 (91, 61) -> (89, 61)
  line L783 (89, 61) -> (89, 59)
  line L784 (91, 59) -> (91, 61)
  line L785 (89, 59) -> (91, 59)
  line L786 (99, 59) -> (101, 59)
  line L787 (99, 61) -> (99, 59)
  line L788 (101, 59) -> (101, 61)
  line L789 (101, 61) -> (99, 61)
  line L790 (11, 61) -> (9, 61)
  line L791 (1, 61) -> (-1, 61)
  line L792 (1, 59) -> (1, 61)
  line L793 (9, 61) -> (9, 59)
  line L794 (11, 59) -> (11, 61)
  line L795 (9, 59) -> (11, 59)
  line L796 (-1, 61) -> (-1, 59)
  line L797 (-1, 59) -> (1, 59)
  line L798 (21, 61) -> (19, 61)
  line L799 (19, 61) -> (19, 59)
  line L800 (21, 59) -> (21, 61)
  line L801 (19, 59) -> (21, 59)
  line L802 (0, 185) -> (0, -64.2875)
  line L803 (51, 71) -> (49, 71)
  line L804 (49, 71) -> (49, 69)
  line L805 (49, 69) -> (51, 69)
  line L806 (61, 71) -> (59, 71)
  line L807 (59, 69) -> (61, 69)
  line L808 (61, 69) -> (61, 71)
  line L809 (59, 71) -> (59, 69)
  line L810 (51, 69) -> (51, 71)
  line L811 (31, 71) -> (29, 71)
  line L812 (29, 71) -> (29, 69)
  line L813 (29, 69) -> (31, 69)
  line L814 (31, 69) -> (31, 71)
  line L815 (41, 71) -> (39, 71)
  line L816 (39, 71) -> (39, 69)
  line L817 (41, 69) -> (41, 71)
  line L818 (39, 69) -> (41, 69)
  line L819 (71, 71) -> (69, 71)
  line L820 (69, 71) -> (69, 69)
  line L821 (71, 69) -> (71, 71)
  line L822 (69, 69) -> (71, 69)
  line L823 (79, 69) -> (81, 69)
  line L824 (79, 71) -> (79, 69)
  line L825 (81, 69) -> (81, 71)
  line L826 (81, 71) -> (79, 71)
  line L827 (91, 71) -> (89, 71)
  line L828 (89, 71) -> (89, 69)
  line L829 (91, 69) -> (91, 71)
  line L830 (89, 69) -> (91, 69)
  line L831 (99, 69) -> (101, 69)
  line L832 (99, 71) -> (99, 69)
  line L833 (101, 69) -> (101, 71)
  line L834 (101, 71) -> (99, 71)
  line L835 (11, 71) -> (9, 71)
  line L836 (1, 71) -> (-1, 71)
  line L837 (1, 69) -> (1, 71)
  line L838 (9, 71) -> (9, 69)
  line L839 (11, 69) -> (11, 71)
  line L840 (9, 69) -> (11, 69)
  line L841 (-1, 71) -> (-1, 69)
  line L842 (-1, 69) -> (1, 69)
  line L843 (21, 71) -> (19, 71)
  line L844 (19, 71) -> (19, 69)
  line L845 (21, 69) -> (21, 71)
  line L846 (19, 69) -> (21, 69)
  line L847 (0, 195) -> (0, -54.2875)
  line L848 (51, 81) -> (49, 81)
  line L849 (49, 81) -> (49, 79)
  line L850 (49, 79) -> (51, 79)
  line L851 (61, 81) -> (59, 81)
  line L852 (59, 79) -> (61, 79)
  line L853 (61, 79) -> (61, 81)
  line L854 (59, 81) -> (59, 79)
  line L855 (51, 79) -> (51, 81)
  line L856 (31, 81) -> (29, 81)
  line L857 (29, 81) -> (29, 79)
  line L858 (29, 79) -> (31, 79)
  line L859 (31, 79) -> (31, 81)
  line L860 (41, 81) -> (39, 81)
  line L861 (39, 81) -> (39, 79)
  line L862 (41, 79) -> (41, 81)
  line L863 (39, 79) -> (41, 79)
  line L864 (71, 81) -> (69, 81)
  line L865 (69, 81) -> (69, 79)
  line L866 (71, 79) -> (71, 81)
  line L867 (69, 79) -> (71, 79)
  line L868 (79, 79) -> (81, 79)
  line L869 (79, 81) -> (79, 79)
  line L870 (81, 79) -> (81, 81)
  line L871 (81, 81) -> (79, 81)
  line L872 (91, 81) -> (89, 81)
  line L873 (89, 81) -> (89, 79)
  line L874 (91, 79) -> (91, 81)
  line L875 (89, 79) -> (91, 79)
  line L876 (99, 79) -> (101, 79)
  line L877 (99, 81) -> (99, 79)
  line L878 (101, 79) -> (101, 81)
  line L879 (101, 81) -> (99, 81)
  line L880 (11, 81) -> (9, 81)
  line L881 (1, 81) -> (-1, 81)
  line L882 (1, 79) -> (1, 81)
  line L883 (9, 81) -> (9, 79)
  line L884 (11, 79) -> (11, 81)
  line L885 (9, 79) -> (11, 79)
  line L886 (-1, 81) -> (-1, 79)
  line L887 (-1, 79) -> (1, 79)
  line L888 (21, 81) -> (19, 81)
  line L889 (19, 81) -> (19, 79)
  line L890 (21, 79) -> (21, 81)
  line L891 (19, 79) -> (21, 79)
  line L892 (0, 205) -> (0, -44.2875)
  line L893 (51, 91) -> (49, 91)
  line L894 (49, 91) -> (49, 89)
  line L895 (49, 89) -> (51, 89)
  line L896 (61, 91) -> (59, 91)
  line L897 (59, 89) -> (61, 89)
  line L898 (61, 89) -> (61, 91)
  line L899 (59, 91) -> (59, 89)
  line L900 (51, 89) -> (51, 91)
  line L901 (31, 91) -> (29, 91)
  line L902 (29, 91) -> (29, 89)
  line L903 (29, 89) -> (31, 89)
  line L904 (31, 89) -> (31, 91)
  line L905 (41, 91) -> (39, 91)
  line L906 (39, 91) -> (39, 89)
  line L907 (41, 89) -> (41, 91)
  line L908 (39, 89) -> (41, 89)
  line L909 (71, 91) -> (69, 91)
  line L910 (69, 91) -> (69, 89)
  line L911 (71, 89) -> (71, 91)
  line L912 (69, 89) -> (71, 89)
  line L913 (79, 89) -> (81, 89)
  line L914 (79, 91) -> (79, 89)
  line L915 (81, 89) -> (81, 91)
  line L916 (81, 91) -> (79, 91)
  line L917 (91, 91) -> (89, 91)
  line L918 (89, 91) -> (89, 89)
  line L919 (91, 89) -> (91, 91)
  line L920 (89, 89) -> (91, 89)
  line L921 (99, 89) -> (101, 89)
  line L922 (99, 91) -> (99, 89)
  line L923 (101, 89) -> (101, 91)
  line L924 (101, 91) -> (99, 91)
  line L925 (11, 91) -> (9, 91)
  line L926 (1, 91) -> (-1, 91)
  line L927 (1, 89) -> (1, 91)
  line L928 (9, 91) -> (9, 89)
  line L929 (11, 89) -> (11, 91)
  line L930 (9, 89) -> (11, 89)
  line L931 (-1, 91) -> (-1, 89)
  line L932 (-1, 89) -> (1, 89)
  line L933 (21, 91) -> (19, 91)
  line L934 (19, 91) -> (19, 89)
  line L935 (21, 89) -> (21, 91)
  line L936 (19, 89) -> (21, 89)
  line L937 (0, 215) -> (0, -34.2875)
  line L938 (51, 101) -> (49, 101)
  line L939 (49, 101) -> (49, 99)
  line L940 (49, 99) -> (51, 99)
  line L941 (61, 101) -> (59, 101)
  line L942 (59, 99) -> (61, 99)
  line L943 (61, 99) -> (61, 101)
  line L944 (59, 101) -> (59, 99)
  line L945 (51, 99) -> (51, 101)
  line L946 (31, 101) -> (29, 101)
  line L947 (29, 101) -> (29, 99)
  line L948 (29, 99) -> (31, 99)
  line L949 (31, 99) -> (31, 101)
  line L950 (41, 101) -> (39, 101)
  line L951 (39, 101) -> (39, 99)
  line L952 (41, 99) -> (41, 101)
  line L953 (39, 99) -> (41, 99)
  line L954 (71, 101) -> (69, 101)
  line L955 (69, 101) -> (69, 99)
  line L956 (71, 99) -> (71, 101)
  line L957 (69, 99) -> (71, 99)
  line L958 (79, 99) -> (81, 99)
  line L959 (79, 101) -> (79, 99)
  line L960 (81, 99) -> (81, 101)
  line L961 (81, 101) -> (79, 101)
  line L962 (91, 101) -> (89, 101)
  line L963 (89, 101) -> (89, 99)
  line L964 (91, 99) -> (91, 101)
  line L965 (89, 99) -> (91, 99)
  line L966 (99, 99) -> (101, 99)
  line L967 (99, 101) -> (99, 99)
  line L968 (101, 99) -> (101, 101)
  line L969 (101, 101) -> (99, 101)
  line L970 (11, 101) -> (9, 101)
  line L971 (1, 101) -> (-1, 101)
  line L972 (1, 99) -> (1, 101)
  line L973 (9, 101) -> (9, 99)
  line L974 (11, 99) -> (11, 101)
  line L975 (9, 99) -> (11, 99)
  line L976 (-1, 101) -> (-1, 99)
  line L977 (-1, 99) -> (1, 99)
  line L978 (21, 101) -> (19, 101)
  line L979 (19, 101) -> (19, 99)
  line L980 (21, 99) -> (21, 101)
  line L981 (19, 99) -> (21, 99)
  line L982 (0, 225) -> (0, -24.2875)
  line L983 (-1, -1) -> (1, -1)
  line L984 (1, 1) -> (-1, 1)
  line L985 (1, -1) -> (1, 1)
  line L986 (-1, 21) -> (-1, 19)
  line L987 (-1, 39) -> (1, 39)
  line L988 (-1, 1) -> (-1, -1)
  line L989 (-1, 71) -> (-1, 69)
  line L990 (1, 69) -> (1, 71)
  line L991 (1, 61) -> (-1, 61)
  line L992 (1, 71) -> (-1, 71)
  line L993 (1, 81) -> (-1, 81)
  line L994 (-1, 81) -> (-1, 79)
  line L995 (-1, 79) -> (1, 79)
  line L996 (1, 79) -> (1, 81)
  line L997 (-1, 91) -> (-1, 89)
  line L998 (-1, 99) -> (1, 99)
  line L999 (1, 89) -> (1, 91)
  line L1000 (1, 99) -> (1, 101)
  line L1001 (-1, 101) -> (-1, 99)
  line L1002 (1, 101) -> (-1, 101)
  line L1003 (1, 91) -> (-1, 91)
  line L1004 (1, -59) -> (-1, -59)
  line L1005 (-1, -59) -> (-1, -61)
  line L1006 (-1, -79) -> (-1, -81)
  line L1007 (1, -69) -> (-1, -69)
  line L1008 (-1, -69) -> (-1, -71)
  line L1009 (-1, -71) -> (1, -71)
  line L1010 (1, -79) -> (-1, -79)
  line L1011 (-1, -81) -> (1, -81)
  line L1012 (1, -71) -> (1, -69)
  line L1013 (1, -91) -> (1, -89)
  line L1014 (1, -89) -> (-1, -89)
  line L1015 (1, 11) -> (-1, 11)
  line L1016 (1, -9) -> (-1, -9)
  line L1017 (-1, -9) -> (-1, -11)
  line L1018 (1, -11) -> (1, -9)
  line L1019 (-1, -11) -> (1, -11)
  line L1020 (1, -19) -> (-1, -19)
  line L1021 (-1, -19) -> (-1, -21)
  line L1022 (1, -21) -> (1, -19)
  line L1023 (-1, -21) -> (1, -21)
  line L1024 (-1, -29) -> (-1, -31)
  line L1025 (1, -31) -> (1, -29)
  line L1026 (-1, -31) -> (1, -31)
  line L1027 (1, -39) -> (-1, -39)
  line L1028 (-1, -39) -> (-1, -41)
  line L1029 (1, -41) -> (1, -39)
  line L1030 (1, -29) -> (-1, -29)
  line L1031 (-1, -41) -> (1, -41)
  line L1032 (-1, -49) -> (-1, -51)
  line L1033 (1, -51) -> (1, -49)
  line L1034 (-1, -51) -> (1, -51)
  line L1035 (-1, -61) -> (1, -61)
  line L1036 (1, -61) -> (1, -59)
  line L1037 (1, -49) -> (-1, -49)
  line L1038 (-1, 41) -> (-1, 39)
  line L1039 (1, 1) -> (-1, 1)
  line L1040 (1, -81) -> (1, -79)
  line L1041 (-1, -89) -> (-1, -91)
  line L1042 (-1, -91) -> (1, -91)
  line L1043 (1, -99) -> (-1, -99)
  line L1044 (-1, -99) -> (-1, -101)
  line L1045 (-1, -101) -> (1, -101)
  line L1046 (1, -101) -> (1, -99)
  line L1047 (1, 21) -> (-1, 21)
  line L1048 (-1, 9) -> (1, 9)
  line L1049 (-1, 11) -> (-1, 9)
  line L1050 (-1, -1) -> (1, -1)
  line L1051 (-1, 1) -> (-1, -1)
  line L1052 (1, -1) -> (1, 1)
  line L1053 (1, 9) -> (1, 11)
  line L1054 (1, 59) -> (1, 61)
  line L1055 (-1, 59) -> (1, 59)
  line L1056 (-1, 61) -> (-1, 59)
  line L1057 (1, 49) -> (1, 51)
  line L1058 (1, 51) -> (-1, 51)
  line L1059 (-1, 49) -> (1, 49)
  line L1060 (-1, 51) -> (-1, 49)
  line L1061 (1, 41) -> (-1, 41)
  line L1062 (1, 39) -> (1, 41)
  line L1063 (1, 19) -> (1, 21)
  line L1064 (-1, 19) -> (1, 19)
  line L1065 (1, 31) -> (-1, 31)
  line L1066 (-1, 31) -> (-1, 29)
  line L1067 (1, 29) -> (1, 31)
  line L1068 (-1, 29) -> (1, 29)
  line L1069 (-1, 69) -> (1, 69)
  line L1070 (-1, 89) -> (1, 89)
  line L1071 (-11, -1) -> (-9, -1)
  line L1072 (-9, 1) -> (-11, 1)
  line L1073 (-9, -1) -> (-9, 1)
  line L1074 (-11, 21) -> (-11, 19)
  line L1075 (-11, 39) -> (-9, 39)
  line L1076 (-11, 1) -> (-11, -1)
  line L1077 (-11, 71) -> (-11, 69)
  line L1078 (-9, 69) -> (-9, 71)
  line L1079 (-9, 61) -> (-11, 61)
  line L1080 (-9, 71) -> (-11, 71)
  line L1081 (-9, 81) -> (-11, 81)
  line L1082 (-11, 81) -> (-11, 79)
  line L1083 (-11, 79) -> (-9, 79)
  line L1084 (-9, 79) -> (-9, 81)
  line L1085 (-11, 91) -> (-11, 89)
  line L1086 (-11, 99) -> (-9, 99)
  line L1087 (-9, 89) -> (-9, 91)
  line L1088 (-9, 99) -> (-9, 101)
  line L1089 (-11, 101) -> (-11, 99)
  line L1090 (-9, 101) -> (-11, 101)
  line L1091 (-9, 91) -> (-11, 91)
  line L1092 (-9, -59) -> (-11, -59)
  line L1093 (-11, -59) -> (-11, -61)
  line L1094 (-11, -79) -> (-11, -81)
  line L1095 (-9, -69) -> (-11, -69)
  line L1096 (-11, -69) -> (-11, -71)
  line L1097 (-11, -71) -> (-9, -71)
  line L1098 (-9, -79) -> (-11, -79)
  line L1099 (-11, -81) -> (-9, -81)
  line L1100 (-9, -71) -> (-9, -69)
  line L1101 (-9, -91) -> (-9, -89)
  line L1102 (-9, -89) -> (-11, -89)
  line L1103 (-9, 11) -> (-11, 11)
  line L1104 (-9, -9) -> (-11, -9)
  line L1105 (-11, -9) -> (-11, -11)
  line L1106 (-9, -11) -> (-9, -9)
  line L1107 (-11, -11) -> (-9, -11)
  line L1108 (-9, -19) -> (-11, -19)
  line L1109 (-11, -19) -> (-11, -21)
  line L1110 (-9, -21) -> (-9, -19)
  line L1111 (-11, -21) -> (-9, -21)
  line L1112 (-11, -29) -> (-11, -31)
  line L1113 (-9, -31) -> (-9, -29)
  line L1114 (-11, -31) -> (-9, -31)
  line L1115 (-9, -39) -> (-11, -39)
  line L1116 (-11, -39) -> (-11, -41)
  line L1117 (-9, -41) -> (-9, -39)
  line L1118 (-9, -29) -> (-11, -29)
  line L1119 (-11, -41) -> (-9, -41)
  line L1120 (-11, -49) -> (-11, -51)
  line L1121 (-9, -51) -> (-9, -49)
  line L1122 (-11, -51) -> (-9, -51)
  line L1123 (-11, -61) -> (-9, -61)
  line L1124 (-9, -61) -> (-9, -59)
  line L1125 (-9, -49) -> (-11, -49)
  line L1126 (-11, 41) -> (-11, 39)
  line L1127 (-9, 1) -> (-11, 1)
  line L1128 (-9, -81) -> (-9, -79)
  line L1129 (-11, -89) -> (-11, -91)
  line L1130 (-11, -91) -> (-9, -91)
  line L1131 (-9, -99) -> (-11, -99)
  line L1132 (-11, -99) -> (-11, -101)
  line L1133 (-11, -101) -> (-9, -101)
  line L1134 (-9, -101) -> (-9, -99)
  line L1135 (-9, 21) -> (-11, 21)
  line L1136 (-11, 9) -> (-9, 9)
  line L1137 (-11, 11) -> (-11, 9)
  line L1138 (-11, -1) -> (-9, -1)
  line L1139 (-11, 1) -> (-11, -1)
  line L1140 (-9, -1) -> (-9, 1)
  line L1141 (-9, 9) -> (-9, 11)
  line L1142 (-9, 59) -> (-9, 61)
  line L1143 (-11, 59) -> (-9, 59)
  line L1144 (-11, 61) -> (-11, 59)
  line L1145 (-9, 49) -> (-9, 51)
  line L1146 (-9, 51) -> (-11, 51)
  line L1147 (-11, 49) -> (-9, 49)
  line L1148 (-11, 51) -> (-11, 49)
  line L1149 (-9, 41) -> (-11, 41)
  line L1150 (-9, 39) -> (-9, 41)
  line L1151 (-9, 19) -> (-9, 21)
  line L1152 (-11, 19) -> (-9, 19)
  line L1153 (-9, 31) -> (-11, 31)
  line L1154 (-11, 31) -> (-11, 29)
  line L1155 (-9, 29) -> (-9, 31)
  line L1156 (-11, 29) -> (-9, 29)
  line L1157 (-11, 69) -> (-9, 69)
  line L1158 (-11, 89) -> (-9, 89)
  line L1159 (-21, -1) -> (-19, -1)
  line L1160 (-19, 1) -> (-21, 1)
  line L1161 (-19, -1) -> (-19, 1)
  line L1162 (-21, 21) -> (-21, 19)
  line L1163 (-21, 39) -> (-19, 39)
  line L1164 (-21, 1) -> (-21, -1)
  line L1165 (-21, 71) -> (-21, 69)
  line L1166 (-19, 69) -> (-19, 71)
  line L1167 (-19, 61) -> (-21, 61)
  line L1168 (-19, 71) -> (-21, 71)
  line L1169 (-19, 81) -> (-21, 81)
  line L1170 (-21, 81) -> (-21, 79)
  line L1171 (-21, 79) -> (-19, 79)
  line L1172 (-19, 79) -> (-19, 81)
  line L1173 (-21, 91) -> (-21, 89)
  line L1174 (-21, 99) -> (-19, 99)
  line L1175 (-19, 89) -> (-19, 91)
  line L1176 (-19, 99) -> (-19, 101)
  line L1177 (-21, 101) -> (-21, 99)
  line L1178 (-19, 101) -> (-21, 101)
  line L1179 (-19, 91) -> (-21, 91)
  line L1180 (-19, -59) -> (-21, -59)
  line L1181 (-21, -59) -> (-21, -61)
  line L1182 (-21, -79) -> (-21, -81)
  line L1183 (-19, -69) -> (-21, -69)
  line L1184 (-21, -69) -> (-21, -71)
  line L1185 (-21, -71) -> (-19, -71)
  line L1186 (-19, -79) -> (-21, -79)
  line L1187 (-21, -81) -> (-19, -81)
  line L1188 (-19, -71) -> (-19, -69)
  line L1189 (-19, -91) -> (-19, -89)
  line L1190 (-19, -89) -> (-21, -89)
  line L1191 (-19, 11) -> (-21, 11)
  line L1192 (-19, -9) -> (-21, -9)
  line L1193 (-21, -9) -> (-21, -11)
  line L1194 (-19, -11) -> (-19, -9)
  line L1195 (-21, -11) -> (-19, -11)
  line L1196 (-19, -19) -> (-21, -19)
  line L1197 (-21, -19) -> (-21, -21)
  line L1198 (-19, -21) -> (-19, -19)
  line L1199 (-21, -21) -> (-19, -21)
  line L1200 (-21, -29) -> (-21, -31)
  line L1201 (-19, -31) -> (-19, -29)
  line L1202 (-21, -31) -> (-19, -31)
  line L1203 (-19, -39) -> (-21, -39)
  line L1204 (-21, -39) -> (-21, -41)
  line L1205 (-19, -41) -> (-19, -39)
  line L1206 (-19, -29) -> (-21, -29)
  line L1207 (-21, -41) -> (-19, -41)
  line L1208 (-21, -49) -> (-21, -51)
  line L1209 (-19, -51) -> (-19, -49)
  line L1210 (-21, -51) -> (-19, -51)
  line L1211 (-21, -61) -> (-19, -61)
  line L1212 (-19, -61) -> (-19, -59)
  line L1213 (-19, -49) -> (-21, -49)
  line L1214 (-21, 41) -> (-21, 39)
  line L1215 (-19, 1) -> (-21, 1)
  line L1216 (-19, -81) -> (-19, -79)
  line L1217 (-21, -89) -> (-21, -91)
  line L1218 (-21, -91) -> (-19, -91)
  line L1219 (-19, -99) -> (-21, -99)
  line L1220 (-21, -99) -> (-21, -101)
  line L1221 (-21, -101) -> (-19, -101)
  line L1222 (-19, -101) -> (-19, -99)
  line L1223 (-19, 21) -> (-21, 21)
  line L1224 (-21, 9) -> (-19, 9)
  line L1225 (-21, 11) -> (-21, 9)
  line L1226 (-21, -1) -> (-19, -1)
  line L1227 (-21, 1) -> (-21, -1)
  line L1228 (-19, -1) -> (-19, 1)
  line L1229 (-19, 9) -> (-19, 11)
  line L1230 (-19, 59) -> (-19, 61)
  line L1231 (-21, 59) -> (-19, 59)
  line L1232 (-21, 61) -> (-21, 59)
  line L1233 (-19, 49) -> (-19, 51)
  line L1234 (-19, 51) -> (-21, 51)
  line L1235 (-21, 49) -> (-19, 49)
  line L1236 (-21, 51) -> (-21, 49)
  line L1237 (-19, 41) -> (-21, 41)
  line L1238 (-19, 39) -> (-19, 41)
  line L1239 (-19, 19) -> (-19, 21)
  line L1240 (-21, 19) -> (-19, 19)
  line L1241 (-19, 31) -> (-21, 31)
  line L1242 (-21, 31) -> (-21, 29)
  line L1243 (-19, 29) -> (-19, 31)
  line L1244 (-21, 29) -> (-19, 29)
  line L1245 (-21, 69) -> (-19, 69)
  line L1246 (-21, 89) -> (-19, 89)
  point P0 (0, 0)
  dimension "d24" = 2
  dimension "d25" = 2
  dimension "d28" = 10
  dimension "d31" = 10
  dimension "d36" = 10
  dimension "d43" = 10
  constraints: 2494 end point, 4 horizontal, 3 vertical, 2 midpoint, 2 parallel, 1 collinear, 1 perpendicular, 2488 other
  measures "d24" distance of L2.end L1.end
  measures "d25" distance of L1.end L0.end
  measures "d28" distance of L1.end L8.start
  measures "d31" distance of L1.end L48.start
  measures "d36" distance of L68.start L488.start
  measures "d43" distance of L10.start L983.end
extrude "Extrusion2" cut sketch "Sketch2" against normal blind 10
sketch "Sketch3" plane through (0, 5, 0) normal (0, 1, 0) x (1, 0, 0)
  line L0 (25, 0) -> (46.6506, -12.5)
  line L1 (25, 0) -> (50, 0) construction
  arc A0 (46.6506, -12.5) -> (50, 0) centre (48.9231, -6.4102) ccw
  line L2 (46.6506, -12.5) -> (50, 0) construction
  line L3 (46.6506, -12.5) -> (59.5916, -12.5) construction
  line L4 (21, 0) -> (55.2016, 0)
  line L5 (25, 0) -> (46.6506, 12.5)
  arc A1 (50, 0) -> (46.6506, 12.5) centre (48.9231, 6.4102) ccw
  point P0 (0, 0)
  dimension "d50" = 25
  dimension "d51" = 30
  dimension "d52" = 75
  dimension "d53" = 6.5
  constraints: 12 end point, 4 point on circle, 3 horizontal, 2 centre point, 2 equal length, 2 symmetric about line, 1 other
  measures "d50" distance of L0.start L0.end
  measures "d51" angle of L0 L1
  measures "d52" angle of L3 L2
  measures "d53" radius of A0
extrude "Extrusion3" cut sketch "Sketch3" against normal blind 10
body "Solid1"
